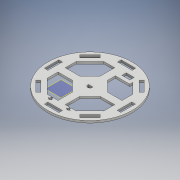
# Autodesk Inventor part: Positioner_Fija_BASE
Saved by Autodesk Inventor 2018 (Build 220112000, 112)
## iProperties
Created: 2017-08-06
Part Number: Positioner_Fija_BASE
Material: Generic
Document SubType Name: Sheet Metal
Designer: Bardo91
Density: 1 g/cm^3
Sheet Metal Rule: Default_mm
Appearance: Default
Author: Bardo91
Autodesk Inventor part; units mm, degrees
ref_plane "YZ Plane" through (0, 0, 0) normal (1, 0, 0) x (0, 1, 0)
ref_plane "XZ Plane" through (0, 0, 0) normal (0, 1, 0) x (-1, 0, 0)
ref_plane "XY Plane" through (0, 0, 0) normal (0, 0, 1) x (1, 0, 0)
sketch "Sketch8" plane through (0, 0, 0) normal (0, 0, 1) x (1, 0, 0)
  circle A0 centre (20, 20) radius 58
  point P0 (0, 0)
  dimension "d48" = 116
  constraints: 1 centre point
  measures "d48" diameter of A0
ref_plane "Work Plane2" through (0, 0, 0) normal (0, 0, -1) x (-1, 0, 0)
sketch "Sketch9" plane through (0, 0, 0) normal (0, 0, -1) x (-1, 0, 0)
  line L0 (0, 40) -> (0, 0) projected
  line L1 (0, 20) -> (-20, 20)
  circle A0 centre (-20, 20) radius 7.375
  dimension "d39" = 20
  dimension "d40" = 14.75
  constraints: 2 end point, 1 centre point, 1 coincident, 1 horizontal, 1 midpoint
  measures "d39" distance of L1.start L1.end
  measures "d40" diameter of A0
extrude "Extrusion9" add sketch "Sketch9" along normal blind 6
sketch "Sketch10" plane through (20, 20, -6) normal (0, 0, -1) x (-1, 0, 0)
  circle A0 centre (0, 0) radius 3.125
  line L0 (0, 0) -> (0, 1)
  line L1 (0, 1) -> (-2.9607, 1)
  line L2 (0, 1) -> (2.9607, 1)
  point P0 (20, -20)
  dimension "d43" = 6.25
  dimension "d44" = 1
  constraints: 6 end point, 2 point on circle, 1 centre point, 1 perpendicular, 1 point on line, 1 vertical
  measures "d43" diameter of A0
  measures "d44" distance of L0.start L0.end
extrude "Extrusion10" cut sketch "Sketch10" against normal blind 15 contours A0 L1 L2 picked at (-0.0807, -1.7325)
extrude "Extrusion12" add sketch "Sketch8" along normal blind 3
sketch "Sketch11" plane through (0, 0, 0) normal (0, 0, -1) x (-1, 0, 0)
  arc A0 (-22.9607, 21) -> (-17.0393, 21) centre (-20, 20) ccw projected
  line L0 (-22.9607, 21) -> (-17.0393, 21) projected
  line L1 (-17.0393, 21) -> (-17.0393, 21)
  arc A1 (-22.9607, 21) -> (-17.0393, 21) centre (-20, 20) ccw
  circle A2 centre (-20, 20) radius 58 projected
  line L2 (-20, 20) -> (38, 20) construction
  line L3 (13.9411, 53.9411) -> (17.4767, 57.4767)
  line L4 (17.4767, 57.4767) -> (10.4056, 64.5477)
  line L5 (10.4056, 64.5477) -> (6.8701, 61.0122)
  line L6 (6.8701, 61.0122) -> (13.9411, 53.9411)
  line L7 (13.9411, 53.9411) -> (21.0122, 46.8701)
  line L8 (21.0122, 46.8701) -> (24.5477, 50.4056)
  line L9 (24.5477, 50.4056) -> (17.4767, 57.4767)
  line L10 (-20, 73) -> (-10, 73)
  line L11 (-10, 73) -> (-10, 68)
  line L12 (-10, 68) -> (-30, 68)
  line L13 (-30, 68) -> (-30, 73)
  line L14 (-30, 73) -> (-20, 73)
  line L15 (-57.4767, 57.4767) -> (-50.4056, 64.5477)
  line L16 (-50.4056, 64.5477) -> (-46.8701, 61.0122)
  line L17 (-46.8701, 61.0122) -> (-61.0122, 46.8701)
  line L18 (-61.0122, 46.8701) -> (-64.5477, 50.4056)
  line L19 (-64.5477, 50.4056) -> (-57.4767, 57.4767)
  line L20 (-72.6799, 20) -> (-72.6799, 30)
  line L21 (-72.6799, 30) -> (-67.6799, 30)
  line L22 (-67.6799, 30) -> (-67.6799, 10)
  line L23 (-67.6799, 10) -> (-72.6799, 10)
  line L24 (-72.6799, 10) -> (-72.6799, 20)
  line L25 (-57.4767, -17.4767) -> (-64.5477, -10.4056)
  line L26 (-64.5477, -10.4056) -> (-61.0122, -6.8701)
  line L27 (-61.0122, -6.8701) -> (-46.8701, -21.0122)
  line L28 (-46.8701, -21.0122) -> (-50.4056, -24.5477)
  line L29 (-50.4056, -24.5477) -> (-57.4767, -17.4767)
  line L30 (-20, -33) -> (-10, -33)
  line L31 (-10, -33) -> (-10, -28)
  line L32 (-10, -28) -> (-30, -28)
  line L33 (-30, -28) -> (-30, -33)
  line L34 (-30, -33) -> (-20, -33)
  line L35 (17.4767, -17.4767) -> (24.5477, -10.4056)
  line L36 (24.5477, -10.4056) -> (21.0122, -6.8701)
  line L37 (21.0122, -6.8701) -> (6.8701, -21.0122)
  line L38 (6.8701, -21.0122) -> (10.4056, -24.5477)
  line L39 (10.4056, -24.5477) -> (17.4767, -17.4767)
  line L40 (33, 20) -> (33, 30)
  line L41 (33, 30) -> (28, 30)
  line L42 (28, 30) -> (28, 10)
  line L43 (28, 10) -> (33, 10)
  line L44 (33, 10) -> (33, 20)
  line L45 (-25, 15) -> (-32.0711, 7.9289)
  line L46 (-32.0711, 7.9289) -> (-25, 0.8579)
  line L47 (-25, 0.8579) -> (-25, -19.1421)
  line L48 (-32.0711, 7.9289) -> (-39.1421, 15)
  line L49 (-39.1421, 15) -> (-59.1421, 15)
  line L50 (-59.1421, 15) -> (-59.1421, 0)
  line L51 (-59.1421, 0) -> (-49.5711, -9.5711)
  line L52 (-25, -19.1421) -> (-40, -19.1421)
  line L53 (-40, -19.1421) -> (-49.5711, -9.5711)
  line L54 (-7.9289, 32.0711) -> (-0.8579, 25)
  line L55 (-0.8579, 25) -> (19.1421, 25)
  line L56 (-7.9289, 32.0711) -> (-15, 39.1421)
  line L57 (-15, 39.1421) -> (-15, 59.1421)
  line L58 (-15, 59.1421) -> (0, 59.1421)
  line L59 (0, 59.1421) -> (9.5711, 49.5711)
  line L60 (19.1421, 25) -> (19.1421, 40)
  line L61 (19.1421, 40) -> (9.5711, 49.5711)
  line L62 (-20, 20) -> (-78, 20) construction
  line L63 (-25, 39.1421) -> (-25, 59.1421)
  line L64 (-25, 59.1421) -> (-40, 59.1421)
  line L65 (-40, 59.1421) -> (-49.5711, 49.5711)
  line L66 (-59.1421, 40) -> (-49.5711, 49.5711)
  line L67 (-59.1421, 25) -> (-59.1421, 40)
  line L68 (-39.1421, 25) -> (-59.1421, 25)
  line L69 (-32.0711, 32.0711) -> (-39.1421, 25)
  line L70 (-32.0711, 32.0711) -> (-25, 39.1421)
  line L71 (-7.9289, 7.9289) -> (-15, 0.8579)
  line L72 (-15, 0.8579) -> (-15, -19.1421)
  line L73 (-7.9289, 7.9289) -> (-0.8579, 15)
  line L74 (-0.8579, 15) -> (19.1421, 15)
  line L75 (19.1421, 15) -> (19.1421, 0)
  line L76 (19.1421, 0) -> (9.5711, -9.5711)
  line L77 (-15, -19.1421) -> (0, -19.1421)
  line L78 (0, -19.1421) -> (9.5711, -9.5711)
  point P0 (0, 0)
  dimension "d55" = 10
  dimension "d56" = 10
  dimension "d58" = 10
  dimension "d59" = 5
  dimension "d60" = 20
  dimension "d62" = 10
  dimension "d63" = 5
  dimension "d64" = 20
  dimension "d67" = 5
  dimension "d68" = 5
  dimension "d69" = 5
  dimension "d70" = 20
  dimension "d71" = 10
  dimension "d72" = 10
  dimension "d73" = 20
  dimension "d74" = 10
  dimension "d75" = 20
  dimension "d76" = 15
  dimension "d77" = 15
  constraints: 156 end point, 32 perpendicular, 18 point on line, 2 horizontal, 2 point on circle, 1 centre point, 1 coincident, 1 collinear, 1 vertical
  measures "d55" distance of L3.end L4.end
  measures "d56" distance of L3.start L7.end
  measures "d58" distance of L10.start L10.end
  measures "d59" distance of L10.end L11.end
  measures "d60" distance of L11.end L12.end
  measures "d62" distance of L20.start L20.end
  measures "d63" distance of L20.end L21.end
  measures "d64" distance of L21.end L22.end
  measures "d67" distance of L30.end L31.end
  measures "d68" distance of L2.end L40.start
  measures "d69" distance of L40.end L41.end
  measures "d70" distance of L41.end L42.end
  measures "d71" distance of L45.start L45.end
  measures "d72" distance of L45.end L46.end
  measures "d73" distance of L46.end L47.end
  measures "d74" distance of L45.end L48.end
  measures "d75" distance of L48.end L49.end
  measures "d76" distance of L49.end L50.end
  measures "d77" distance of L47.end L52.end
extrude "Extrusion13" cut sketch "Sketch11" against normal blind 3 contours L0 A0 | L6 L5 L4 L3 | L3 L9 L8 L7 | L10 L11 L12 L13 L14 | L15 L16 L17 L18 L19 | L20 L21 L22 L23 L24 | L25 L26 L27 L28 L29 | L34 L33 L32 L31 L30 | L39 L38 L37 L36 L35 | L44 L43 L42 L41 L40 | L46 L47 L52 L53 L51 L50 L49 L48 | L56 L57 L58 L59 L61 L60 L55 L54 | L70 L69 L68 L67 L66 L65 L64 L63 | L73 L74 L75 L76 L78 L77 L72 L71
fillet "Fillet2" radius 0.5 2 edges at (20, 16.875, -6) (20, 21, -6)
sketch "Sketch12" plane through (20, 20, 0) normal (0, 0, -1) x (-1, 0, 0)
  line L0 (0, 40) -> (-20, 40)
  line L1 (-20, 40) -> (-20, 35)
  line L2 (-20, 35) -> (0, 35)
  line L3 (0, 35) -> (0, 40)
  line L4 (0, 40) -> (0, 43)
  line L5 (0, 43) -> (-23, 43)
  line L6 (-23, 43) -> (-23, 30)
  line L7 (-23, 30) -> (0, 30)
  line L8 (0, 30) -> (0, 35)
  point P0 (20, -20)
  dimension "d82" = 20
  dimension "d83" = 5
  dimension "d84" = 3
  dimension "d85" = 23
  dimension "d86" = 13
  constraints: 18 end point, 5 perpendicular, 2 vertical, 1 horizontal, 1 point on line
  measures "d82" distance of L0.start L0.end
  measures "d83" distance of L0.end L1.end
  measures "d84" distance of L0.start L4.end
  measures "d85" distance of L4.end L5.end
  measures "d86" distance of L5.end L6.end
extrude "Extrusion14" add sketch "Sketch12" against normal blind 3 contours L0 L1 L2 L8 L7 L6 L5 L4
sketch "Sketch13" plane through (20, 20, 0) normal (0, 0, -1) x (-1, 0, 0)
  line L0 (-5, 35) -> (-20, 35) projected
  line L1 (-20, 35) -> (-20, 39.1421) projected
  line L2 (-10, 40) -> (-10, 35)
  line L3 (-5, 39.1421) -> (-5, 35) projected
  line L4 (-10, 35) -> (-5, 35)
  line L5 (-5, 35) -> (-5, 39.1421)
  line L6 (-5, 39.1421) -> (-10, 39.1421)
  line L7 (-20, 39.1421) -> (-5, 39.1421) projected
  point P0 (20, -20)
  constraints: 8 end point, 2 perpendicular, 2 point on line
extrude "Extrusion15" add sketch "Sketch13" against normal blind 3 contours L0 L2 L6 L3
sketch "Sketch14" plane through (20, 20, 0) normal (0, 0, -1) x (-1, 0, 0)
  line L0 (-20, 39.1421) -> (-20, 35) projected
  line L1 (-20, 35) -> (-20, 41)
  line L2 (-20, 41) -> (-9, 41)
  line L3 (-9, 41) -> (-9, 35)
  line L4 (-10, 35) -> (-20, 35) projected
  line L5 (-9, 35) -> (-20, 35)
  point P0 (20, -20)
  dimension "d93" = 6
  dimension "d94" = 11
  constraints: 8 end point, 2 collinear, 2 perpendicular
  measures "d93" distance of L0.end L1.end
  measures "d94" distance of L1.end L2.end
extrude "Extrusion16" cut sketch "Sketch14" against normal blind 3
sketch "Sketch15" plane through (20, 20, 0) normal (0, 0, -1) x (-1, 0, 0)
  line L0 (-23, 30) -> (-5, 30) projected
  line L1 (-23, 30) -> (-25, 30)
  line L2 (-25, 30) -> (-25, 34.1421)
  line L3 (-39.1421, 20) -> (-23, 36.1421) projected
  line L4 (-23, 36.1421) -> (-23, 30)
  point P0 (20, -20)
  dimension "d97" = 2
  constraints: 6 end point, 1 horizontal, 1 parallel, 1 perpendicular, 1 point on line
  measures "d97" distance of L0.start L1.end
extrude "Extrusion17" add sketch "Sketch15" against normal blind 3
sketch "Sketch16" plane through (20, 20, 0) normal (0, 0, -1) x (-1, 0, 0)
  line L0 (-12.5, -39.1421) -> (-13.5, -39.1421)
  line L1 (-13.5, -39.1421) -> (-13.5, -42.1421)
  line L2 (-12.5, -39.1421) -> (-11.5, -39.1421)
  line L3 (-11.5, -39.1421) -> (-11.5, -42.1421)
  line L4 (-11.5, -42.1421) -> (-10.5, -42.1421)
  line L5 (-10.5, -42.1421) -> (-9.5, -42.1421)
  line L6 (-13.5, -42.1421) -> (-15.5, -42.1421)
  line L7 (-15.5, -42.1421) -> (-12.5, -44.1421)
  line L8 (-12.5, -44.1421) -> (-9.5, -42.1421)
  line L9 (12.5529, -39.2173) -> (13.5529, -39.2232)
  line L10 (13.5529, -39.2232) -> (13.5349, -42.2232)
  line L11 (12.5529, -39.2173) -> (11.5529, -39.2113)
  line L12 (11.5529, -39.2113) -> (11.5349, -42.2112)
  line L13 (11.5349, -42.2112) -> (10.5349, -42.2052)
  line L14 (10.5349, -42.2052) -> (9.535, -42.1992)
  line L15 (13.5349, -42.2232) -> (15.5348, -42.2352)
  line L16 (15.5348, -42.2352) -> (12.5229, -44.2172)
  line L17 (12.5229, -44.2172) -> (9.535, -42.1992)
  point P0 (20, -20)
  dimension "d104" = 1
  dimension "d105" = 1
  dimension "d106" = 1
  dimension "d107" = 2
  constraints: 36 end point, 3 perpendicular, 2 point on line, 1 horizontal
  measures "d104" distance of L0.start L2.end
  measures "d105" distance of L3.end L4.end
  measures "d106" distance of L4.end L5.end
  measures "d107" distance of L1.end L6.end
extrude "Extrusion18" cut sketch "Sketch16" against normal blind 3
equation "\"BendRadius\" = Thickness"
equation "\"BendReliefWidth\" = Thickness"
equation "\"BendReliefDepth\" = 0.5 * Thickness"
equation "\"CornerReliefSize\" = 4 * Thickness"
equation "\"MinimumRemnant\" = 2 * Thickness"
equation "\"TransitionRadius\" = BendRadius"
equation "\"JacobiRadiusSize\" = BendRadius"
equation "\"GapSize\" = Thickness"
equation "\"Thickness\" = 0.5"
body "Solid2"
